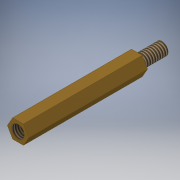
# Autodesk Inventor part: StandoffLong
Saved by Autodesk Inventor 2018 (Build 220112000, 112)
## iProperties
Created: 2018-01-12
Part Number: StandoffLong
Material: Brass, Soft Yellow
Document SubType Name: Modeling
Designer: Kyle
Density: 8.47 g/cm^3
Appearance: Brass - Satin
Author: Kyle
Autodesk Inventor part; units mm, degrees
ref_plane "YZ Plane" through (0, 0, 0) normal (1, 0, 0) x (0, 1, 0)
ref_plane "XZ Plane" through (0, 0, 0) normal (0, 1, 0) x (-1, 0, 0)
ref_plane "XY Plane" through (0, 0, 0) normal (0, 0, 1) x (1, 0, 0)
sketch "Sketch1" plane through (0, 0, 0) normal (0, 0, 1) x (1, 0, 0)
  line L0 (-2.713, 0) -> (-1.3565, 2.3495)
  line L1 (-1.3565, 2.3495) -> (1.3565, 2.3495)
  line L2 (1.3565, 2.3495) -> (2.713, 0)
  line L3 (2.713, 0) -> (1.3565, -2.3495)
  line L4 (1.3565, -2.3495) -> (-1.3565, -2.3495)
  line L5 (-1.3565, -2.3495) -> (-2.713, 0)
  circle A0 centre (0, 0) radius 1.5875
  dimension "d0" = 4.699
  dimension "d1" = 3.175
  constraints: 12 end point, 2 coincident, 1 centre point, 1 horizontal, 13 other
  measures "d0" distance between parallel lines of L4 L1
  measures "d1" diameter of A0
extrude "Extrusion1" add sketch "Sketch1" along normal blind 30.099
sketch "Sketch2" plane through (0, 0, 0) normal (0, 0, -1) x (-1, 0, 0)
  circle A0 centre (0, 0) radius 1.5875
  constraints: 1 centre point, 1 coincident
extrude "Extrusion2" add sketch "Sketch2" along normal blind 6.35
thread "Thread1" size "5-40 UNC" class "2A" standard "ANSI Unified Screw Threads" full length
thread "Thread2" size "5-40 UNC" class "2B" standard "ANSI Unified Screw Threads" full length
body "Solid1"
